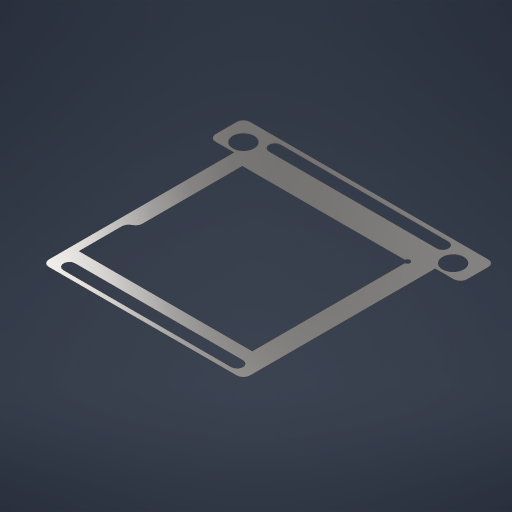
# Autodesk Inventor part: Sensor Mount Film Stencil - V1
Saved by Autodesk Inventor 2024 (Build 280153000, 153)
## iProperties
Created: 2022-06-23
Part Number: Sensor Mount Film Stencil - V1
Material: Stainless Steel
Document SubType Name: Modeling
Designer: Caleb
Density: 8 g/cm^3
Appearance: Semi-Polished
Author: Caleb
Autodesk Inventor part; units mm, degrees
ref_plane "YZ Plane" through (0, 0, 0) normal (1, 0, 0) x (0, 1, 0)
ref_plane "XZ Plane" through (0, 0, 0) normal (0, 1, 0) x (-1, 0, 0)
ref_plane "XY Plane" through (0, 0, 0) normal (0, 0, 1) x (1, 0, 0)
sketch "Sketch1" plane through (0, 0, 0) normal (0, 1, 0) x (-1, 0, 0)
  line L0 (-38.1, -34.29) -> (38.1, -34.29)
  line L1 (38.1, -34.29) -> (38.1, 34.29)
  line L2 (38.1, 34.29) -> (-38.1, 34.29)
  line L3 (-38.1, 34.29) -> (-38.1, -34.29)
  line L4 (-38.1, -34.29) -> (38.1, 34.29) construction
  line L5 (38.1, -34.29) -> (-38.1, 34.29) construction
  point P0 (0, 0)
  dimension "d0" = 76.2
  dimension "d1" = 68.58
  constraints: 12 end point, 2 midpoint, 2 parallel, 1 horizontal, 1 perpendicular
  measures "d0" distance of L2.end L1.end
  measures "d1" distance of L1.end L0.end
extrude "Extrusion1" add sketch "Sketch1" along normal blind 0.0508
sketch "Sketch2" plane through (0, 0.0508, 0) normal (0, 1, 0) x (1, 0, 0)
  line L0 (-38.1, -34.29) -> (38.1, -34.29) projected
  line L1 (-46.3971, 0) -> (43.7494, 0)
  line L2 (-38.1, 34.29) -> (-38.1, -34.29) projected
  line L3 (38.1, -34.29) -> (38.1, 34.29) projected
  line L4 (38.1, 23.79) -> (30.48, 23.79)
  line L5 (30.48, 23.79) -> (30.48, -34.29)
  line L6 (30.48, -34.29) -> (38.1, -34.29)
  line L7 (38.1, -34.29) -> (38.1, 23.79)
  line L8 (0, -45.6355) -> (0, 71.8702)
  line L9 (46.3971, 0) -> (-43.7494, 0)
  line L10 (-38.1, -34.29) -> (-38.1, 34.29)
  line L11 (-38.1, 23.79) -> (-30.48, 23.79)
  line L12 (-30.48, 23.79) -> (-30.48, -34.29)
  line L13 (-30.48, -34.29) -> (-38.1, -34.29)
  line L14 (-38.1, -34.29) -> (-38.1, 23.79)
  line L15 (38.1, 34.29) -> (-38.1, 34.29) projected
  point P0 (0, 0)
  point P1 (38.1, -31.05)
  dimension "d14" = 7.62
  dimension "d16" = 10.5
  constraints: 24 end point, 6 symmetric about line, 3 point on line, 2 horizontal, 2 parallel, 1 perpendicular, 1 vertical
  measures "d14" distance of L5.end L6.end
  measures "d16" distance between parallel lines of L15 L4
extrude "Extrusion2" cut sketch "Sketch2" against normal through all contours L2 L1 L12 L0 | L2 L11 L12 L1 | L5 L1 L3 L0 | L5 L4 L3 L1
sketch "Sketch3" plane through (0, 0.0508, 0) normal (0, 1, 0) x (1, 0, 0)
  line L0 (25.4, -31.115) -> (-25.4, -31.115) construction
  line L1 (25.4, -29.365) -> (-25.4, -29.365)
  line L2 (-25.4, -32.865) -> (25.4, -32.865)
  arc A0 (25.4, -32.865) -> (25.4, -29.365) centre (25.4, -31.115) ccw
  arc A1 (-25.4, -29.365) -> (-25.4, -32.865) centre (-25.4, -31.115) ccw
  line L3 (25.4, 31.115) -> (-25.4, 31.115) construction
  line L4 (25.4, 32.865) -> (-25.4, 32.865)
  line L5 (-25.4, 29.365) -> (25.4, 29.365)
  arc A2 (25.4, 29.365) -> (25.4, 32.865) centre (25.4, 31.115) ccw
  arc A3 (-25.4, 32.865) -> (-25.4, 29.365) centre (-25.4, 31.115) ccw
  line L6 (38.1, 34.29) -> (-38.1, 34.29) projected
  line L7 (-38.1, -34.29) -> (38.1, -34.29) projected
  point P0 (0, 0)
  point P1 (0, -31.115)
  point P2 (0, 31.115)
  dimension "d17" = 3.5
  dimension "d18" = 3.5
  dimension "d19" = 50.8
  dimension "d20" = 50.8
  dimension "d21" = 3.175
  dimension "d22" = 3.175
  constraints: 16 end point, 8 point on circle, 8 tangent, 4 centre point, 3 parallel, 2 midpoint, 2 vertical alignment, 1 horizontal
  measures "d17" distance between parallel lines of L2 L1
  measures "d18" distance between parallel lines of L4 L5
  measures "d19" distance of L0.end L0.start
  measures "d20" distance of L3.end L3.start
  measures "d21" distance from line of L6 point (0, 31.115)
  measures "d22" distance from line of L7 point (0, -31.115)
extrude "Extrusion3" cut sketch "Sketch3" against normal through all
sketch "Sketch6" plane through (0, 0.0508, 0) normal (0, 1, 0) x (1, 0, 0)
  line L0 (38.1, 34.29) -> (-38.1, 34.29) projected
  line L1 (-38.1, 34.29) -> (-38.1, 23.79) projected
  line L2 (38.1, 23.79) -> (38.1, 34.29) projected
  point P0 (0, 0)
  point P1 (-31.75, 27.94)
  point P2 (31.75, 27.94)
  dimension "d41" = 6.35
  dimension "d42" = 6.35
  dimension "d43" = 6.35
  constraints: 1 horizontal alignment
  measures "d41" distance from line of L0 point (-31.75, 27.94)
  measures "d42" distance from line of L1 point (-31.75, 27.94)
  measures "d43" distance from line of point (31.75, 27.94) L2
hole "Hole1" at (-31.75, 0.0508, -27.94) at (31.75, 0.0508, -27.94) direction (0, -1, 0) diameter 6.4262 end through all
sketch "Sketch4" plane through (0, 0.0508, 0) normal (0, 1, 0) x (1, 0, 0)
  line L0 (-25.605, -25.525) -> (24.395, -25.525)
  line L1 (24.395, -25.525) -> (24.395, 21.475)
  line L2 (24.395, 21.475) -> (-25.605, 21.475)
  line L3 (-25.605, 21.475) -> (-25.605, -25.525)
  line L4 (38.1, 34.29) -> (-38.1, 34.29) projected
  line L5 (38.1, 23.79) -> (38.1, 34.29) projected
  circle A0 centre (24.395, 21.475) radius 0.7938
  circle A1 centre (31.75, 27.94) radius 3.2131 projected
  point P0 (0, 0)
  point P1 (24.395, 20.6813)
  point P2 (23.6013, 21.475)
  point P3 (29.845, 22.225)
  dimension "d29" = 1.5875
  dimension "d39" = 47
  dimension "d40" = 50
  dimension "d52" = 1.905
  dimension "d53" = 5.715
  dimension "d54" = 0.75
  dimension "d55" = 5.45
  constraints: 8 end point, 2 parallel, 1 centre point, 1 coincident, 1 horizontal, 1 perpendicular
  measures "d29" diameter of A0
  measures "d39" distance of L2.end L0.start
  measures "d40" distance of L1.end L2.end
  measures "d52" horizontal distance of point (29.845, 22.225) A1.centre
  measures "d53" vertical distance of point (29.845, 22.225) A1.centre
  measures "d54" distance from line of L2 point (29.845, 22.225)
  measures "d55" distance from line of L1 point (29.845, 22.225)
extrude "Extrusion4" cut sketch "Sketch4" against normal through all contours L3 L2 A0 L1 L0 | A0 L2 L1 | L1 L2 A0
sketch "Sketch5" plane through (0, 0.0508, 0) normal (0, 1, 0) x (1, 0, 0)
  line L0 (-25.605, 21.475) -> (-25.605, -25.525) projected
  line L1 (-25.605, -25.525) -> (-28.0425, -25.525)
  line L2 (-28.0425, -25.525) -> (-28.0425, -10.525)
  line L3 (-28.0425, -10.525) -> (-25.605, -10.525)
  line L4 (-25.605, -10.525) -> (-25.605, -25.525)
  line L5 (-30.48, 23.79) -> (-30.48, -34.29) projected
  point P0 (0, 0)
  point P1 (-30.48, -31.05)
  point P2 (-25.605, -10.525)
  dimension "d30" = 15
  dimension "d31" = 4.875
  dimension "d32" = 2.4375
  constraints: 8 end point, 2 parallel, 1 horizontal, 1 perpendicular
  measures "d30" distance of L1.end L2.end
  measures "d31" distance between parallel lines of L5 L0
  measures "d32" distance of L2.end L3.end
extrude "Extrusion5" cut sketch "Sketch5" against normal through all
fillet "Fillet1" radius 2 8 edges at (-38.1, 0.0254, -34.29) (38.1, 0.0254, -34.29) (38.1, 0.0254, -23.79) (-38.1, 0.0254, -23.79) (30.48, 0.0254, 34.29) (-30.48, 0.0254, 34.29) (-25.605, 0.0254, 10.525) (-28.0425, 0.0254, 10.525)
equation "\"d18\" = d17"
equation "\"d20\" = d19"
equation "\"d43\" = d42"
equation "\"d32\" = 0.5 * d31"
body "Solid1"
